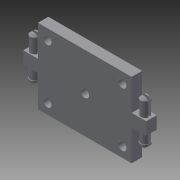
# Autodesk Inventor part: mover01
Saved by Autodesk Inventor 2015 (Build 190159000, 159)
## iProperties
Created: 2016-09-16
Part Number: mover01
Material: Generic
Document SubType Name: Modeling
Designer: spichelh
Density: 1 g/cm^3
Appearance: Default
Author: spichelh
Autodesk Inventor part; units mm, degrees
ref_plane "YZ Plane" through (0, 0, 0) normal (1, 0, 0) x (0, 1, 0)
ref_plane "XZ Plane" through (0, 0, 0) normal (0, 1, 0) x (-1, 0, 0)
sketch "Sketch1" plane through (0, 0, 0) normal (0, 0, 1) x (1, 0, 0)
  line L0 (-22.5, 17.95) -> (22.5, 17.95)
  line L1 (22.5, 17.95) -> (22.5, -17.95)
  line L2 (22.5, -17.95) -> (-22.5, -17.95)
  line L3 (-22.5, -17.95) -> (-22.5, 17.95)
  line L4 (-29.5, 3) -> (29.5, 3)
  line L5 (29.5, 3) -> (29.5, -3)
  line L6 (29.5, -3) -> (-29.5, -3)
  line L7 (-29.5, -3) -> (-29.5, 3)
  line L8 (-22.5, -17.95) -> (22.5, 17.95) construction
  line L9 (-22.5, 17.95) -> (22.5, -17.95) construction
  line L10 (29.5, 3) -> (-29.5, -3) construction
  line L11 (-29.5, 3) -> (29.5, -3) construction
  point P0 (0, 0)
  point P1 (0, 0)
  point P2 (0, 0)
  dimension "d8" = 35.9
  dimension "d9" = 45
  dimension "d10" = 6
  dimension "d11" = 59
  constraints: 24 end point, 6 midpoint, 4 parallel, 2 horizontal, 2 perpendicular
  measures "d8" distance of L2.end L0.start
  measures "d9" distance of L1.end L2.end
  measures "d10" distance of L4.end L5.end
  measures "d11" distance between parallel lines of L5 L7
extrude "Extrusion1" add sketch "Sketch1" along normal blind 5
sketch "Sketch2" plane through (0, 0, 0) normal (0, 0, -1) x (-1, 0, 0)
  circle A0 centre (0, 0) radius 2.05
  circle A1 centre (-18, 13) radius 2
  line L0 (0, 0) -> (16.3137, 0) construction
  line L1 (0, 0) -> (0, -11.5343) construction
  circle A2 centre (18, 13) radius 2
  circle A3 centre (-18, -13) radius 2
  circle A4 centre (18, -13) radius 2
  dimension "d2" = 4
  dimension "d3" = 36
  dimension "d4" = 26
  dimension "d5" = 4.1
  constraints: 5 centre point, 4 end point, 3 symmetric about line, 1 coincident, 1 horizontal, 1 vertical, 3 other
  measures "d2" diameter of A1
  measures "d3" diameter of A1.centre L1
  measures "d4" diameter of A1.centre L0
  measures "d5" diameter of A0
extrude "Extrusion2" cut sketch "Sketch2" against normal blind 5
sketch "Sketch3" plane through (-29.5, 3, 0) normal (0, 1, 0) x (1, 0, 0)
  line L0 (0, 0) -> (0, -5) projected
  line L1 (0, 0) -> (7, 0) projected
  line L2 (1.0635, -2) -> (4.9365, -2)
  line L3 (4.9365, -3) -> (1.0635, -3)
  arc A0 (1.0635, -3) -> (4.9365, -3) centre (3, -2.5) ccw
  arc A1 (4.9365, -2) -> (1.0635, -2) centre (3, -2.5) ccw
  point P0 (29.5, 0)
  dimension "d13" = 3
  dimension "d14" = 2.5
  dimension "d15" = 0.5
  dimension "d16" = 0.5
  dimension "d19" = 2
  dimension "d20" = 2
  constraints: 4 end point, 4 point on circle, 2 centre point, 1 horizontal, 1 parallel
  measures "d13" distance from line of L0 A0.centre
  measures "d14" distance from line of L1 A0.centre
  measures "d15" distance from line of L2 A0.centre
  measures "d16" distance from line of A0.centre L3
  measures "d19" radius of A1
  measures "d20" radius of A0
extrude "Extrusion3" add sketch "Sketch3" along normal blind 6 and the other way blind 11
sketch "Sketch4" plane through (-29.5, 9, 0) normal (0, 1, 0) x (1, 0, 0)
  line L0 (1.0635, -2) -> (4.9365, -2) projected
  arc A0 (4.9365, -2) -> (1.0635, -2) centre (3, -2.5) ccw projected
  line L1 (4.9365, -3) -> (1.0635, -3) projected
  arc A1 (1.0635, -3) -> (4.9365, -3) centre (3, -2.5) ccw projected
  line L2 (1.0635, -1.7) -> (4.9365, -1.7)
  arc A2 (4.9365, -1.7) -> (1.0635, -1.7) centre (3, -2.3) ccw
  line L3 (1.0635, -2) -> (1.0635, -1.7)
  line L4 (4.9365, -1.7) -> (4.9365, -2)
  line L5 (3, -2.5) -> (0.4845, -2.5) construction
  arc A3 (1.0635, -3) -> (4.9365, -3) centre (3, -2.5) ccw
  line L6 (1.0635, -3.3) -> (4.9365, -3.3)
  arc A4 (1.0635, -3.3) -> (4.9365, -3.3) centre (3, -2.7) ccw
  line L7 (1.0635, -3) -> (1.0635, -3.3)
  line L8 (4.9365, -3) -> (4.9365, -3.3)
  point P0 (29.5, 0)
  dimension "d32" = 0.2
  dimension "d33" = 0.3
  constraints: 14 end point, 6 point on circle, 3 centre point, 3 symmetric about line, 3 vertical, 2 horizontal, 2 other
  measures "d32" distance of A0.centre A2.centre
  measures "d33" distance of L2.end L0.end
extrude "Extrusion4" add sketch "Sketch4" along normal blind 2
sketch "Sketch5" plane through (-29.5, -8, 0) normal (0, -1, 0) x (1, 0, 0)
  line L0 (4.9365, 2) -> (1.0635, 2) projected
  arc A0 (1.0635, 2) -> (4.9365, 2) centre (3, 2.5) ccw projected
  line L1 (1.0635, 3) -> (4.9365, 3) projected
  arc A1 (4.9365, 3) -> (1.0635, 3) centre (3, 2.5) ccw projected
  line L2 (4.9365, 1.7) -> (1.0635, 1.7)
  arc A2 (1.0635, 1.7) -> (4.9365, 1.7) centre (3, 2.2) ccw
  line L3 (4.9365, 1.7) -> (4.9365, 2)
  line L4 (1.0635, 2) -> (1.0635, 1.7)
  line L5 (3, 2.5) -> (4.482, 2.5)
  line L6 (4.9365, 3.3) -> (1.0635, 3.3)
  arc A3 (4.9365, 3.3) -> (1.0635, 3.3) centre (3, 2.8) ccw
  line L7 (4.9365, 3.3) -> (4.9365, 3)
  line L8 (1.0635, 3) -> (1.0635, 3.3)
  point P0 (29.5, 0)
  dimension "d35" = 0.3
  dimension "d36" = 0.3
  dimension "d37" = 2
  constraints: 12 end point, 3 symmetric about line, 2 centre point, 2 horizontal, 2 point on circle, 2 vertical, 1 parallel, 1 other
  measures "d35" distance of A0.centre A2.centre
  measures "d36" distance of L0.end L2.end
  measures "d37" radius of A2
extrude "Extrusion5" add sketch "Sketch5" along normal blind 2
sketch "Sketch7" plane through (0, 0, 5) normal (0, 0, 1) x (1, 0, 0)
  circle A0 centre (18, -13) radius 2 projected
  circle A1 centre (-18, 13) radius 2 projected
  circle A2 centre (18, 13) radius 2 projected
  circle A3 centre (-18, -13) radius 2 projected
  circle A4 centre (0, 0) radius 2.05 projected
  line L0 (-22.5, -3) -> (-22.5, -17.95) projected
  line L1 (-22.5, -17.95) -> (22.5, -17.95) projected
  line L2 (22.5, -17.95) -> (22.5, -3) projected
  line L3 (22.5, -3) -> (29.5, -3) projected
  line L4 (29.5, -3) -> (29.5, 3) projected
  line L5 (29.5, 3) -> (22.5, 3) projected
  line L6 (22.5, 3) -> (22.5, 17.95) projected
  line L7 (22.5, 17.95) -> (-22.5, 17.95) projected
  line L8 (-22.5, 17.95) -> (-22.5, 3) projected
  line L9 (-22.5, 3) -> (-29.5, 3) projected
  line L10 (-29.5, 3) -> (-29.5, -3) projected
  line L11 (-29.5, -3) -> (-22.5, -3) projected
ref_plane "Work Plane1" through (0, 0, 5) normal (1, 0, 0) x (0, 0, -1)
mirror "Mirror1" about plane through (0, 0, 5) normal (1, 0, 0) of "Extrusion3", "Extrusion4", "Extrusion5"
chamfer "Chamfer1" distance 1 angle 45 2 edges at (-26.5, 11, 0.2727) (-26.5, 11, 4.7273)
chamfer "Chamfer2" distance 1 angle 45 6 edges at (-26.5, -10, 0.2) (-26.5, -10, 4.8) (26.5, 11, 0.2727) (26.5, 11, 4.7273) (26.5, -10, 0.2) (26.5, -10, 4.8)
body "Solid1"
